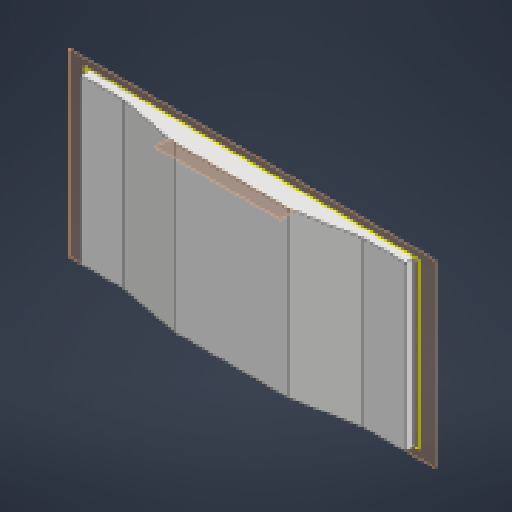
# Autodesk Inventor part: daiza
Saved by Autodesk Inventor 2026.1 (Build 301233020, 233B)
## iProperties
Created: 2026-03-17
Part Number: daiza
Material: 一般
Document SubType Name: Modeling
Designer: kamada
Density: 1 g/cm^3
Appearance: 既定
Author: kamada
Autodesk Inventor part; units mm, degrees
ref_plane "YZ Plane" through (0, 0, 0) normal (1, 0, 0) x (0, 1, 0)
ref_plane "XZ Plane" through (0, 0, 0) normal (0, 1, 0) x (-1, 0, 0)
ref_plane "XY Plane" through (0, 0, 0) normal (0, 0, 1) x (1, 0, 0)
ref_plane "作業平面1" through (0, 0, 0) normal (0, 0, 1) x (1, 0, 0)
ref_plane "作業平面2" through (53.1084, 38.98, 5) normal (0, 1, 0) x (-1, 0, 0)
sketch "スケッチ2" plane through (53.1084, 38.98, 5) normal (0, 1, 0) x (-1, 0, 0)
  line L0 (0, 0) -> (27.0868, 0) projected
  line L1 (27.0868, 0) -> (27.0868, 3) projected
  line L2 (0, 3) -> (27.0868, 3) projected
  line L3 (0, 0) -> (0, 3) projected
  line L4 (53.1084, -5) -> (-26.0192, -5) projected
  line L5 (27.0868, 0) -> (53.1084, -5)
  line L6 (0, 0) -> (-26.0192, -5)
  line L7 (-14.9983, -5) -> (42.0865, -5)
  line L8 (42.0865, -5) -> (42.0865, -2.8822)
  line L9 (42.0865, -2.8822) -> (-14.9983, -2.8822)
  line L10 (-14.9983, -2.8822) -> (-14.9983, -5)
  point P0 (42.0865, -5)
  constraints: 12 end point, 3 point on line, 2 parallel, 1 horizontal, 1 perpendicular
ref_plane "作業平面3" through (-29.3223, 0, -100) normal (0, 1, 0) x (0, 0, 1)
extrude "押し出し1" add sketch "スケッチ2" against normal up to surface (38.98 mm away) contours L0 L5 L9 L6 | L9 L8 L4 L10
sketch "スケッチ3" plane through (68.1068, 38.98, 2.1178) normal (1, 0, 0) x (0, 0, -1)
  line L0 (2.1178, -38.98) -> (0, -38.98) projected
  line L1 (2.1178, 0) -> (2.1178, -38.98) projected
  line L2 (0, 0) -> (2.1178, 0) projected
  line L3 (0, 0) -> (0, -38.98) projected
  point P0 (2.1178, -38.98)
extrude "押し出し2" add sketch "スケッチ3" along normal blind 10
sketch "スケッチ4" plane through (11.0219, 38.98, 0) normal (-1, 0, 0) x (0, 0, 1)
  line L0 (2.1178, -38.98) -> (0, -38.98) projected
  line L1 (2.1178, 0) -> (2.1178, -38.98) projected
  line L2 (0, 0) -> (2.1178, 0) projected
  line L3 (0, 0) -> (0, -38.98) projected
  point P0 (0, -38.98)
extrude "押し出し3" add sketch "スケッチ4" along normal blind 10
sketch "スケッチ5" plane through (78.1068, 0, 0) normal (0, 0, -1) x (-1, 0, 0)
  point P0 (78.1068, 0)
sketch "スケッチ6" plane through (78.1068, 0, 0) normal (0, 0, -1) x (-1, 0, 0)
  line L0 (77.0849, 0) -> (0, 0) projected
  line L1 (44.8216, 0) -> (32.0369, 0)
  line L2 (32.0369, 0) -> (32.0369, 3)
  line L3 (32.0369, 3) -> (44.8216, 3)
  line L4 (44.8216, 3) -> (44.8216, 0)
  point P0 (78.1068, 0)
  dimension "d6" = 3
  constraints: 8 end point, 2 parallel, 1 horizontal, 1 perpendicular, 1 point on line
  measures "d6" distance of L1.end L2.end
extrude "押し出し4" add sketch "スケッチ6" along normal blind 10
sketch "スケッチ7" plane through (26.0216, 0, 5) normal (0, -1, 0) x (1, 0, 0)
  circle A0 centre (13.5428, -12.529) radius 1 projected
  line L0 (-24.9997, -5) -> (7.2636, -5) projected
  line L1 (7.2636, -5) -> (7.2636, -15) projected
  line L2 (20.0483, -15) -> (7.2636, -15) projected
  line L3 (20.0483, -5) -> (20.0483, -15) projected
  line L4 (20.0483, -5) -> (52.0851, -5) projected
  line L5 (52.0851, -2.8822) -> (52.0851, -5) projected
  line L6 (42.0851, -2.8822) -> (52.0851, -2.8822) projected
  line L7 (42.0851, -2.8822) -> (27.0868, 0) projected
  line L8 (27.0868, 0) -> (0, 0) projected
  line L9 (0, 0) -> (-14.9997, -2.8822) projected
  line L10 (-14.9997, -2.8822) -> (-24.9997, -2.8822) projected
  line L11 (-24.9997, -5) -> (-24.9997, -2.8822) projected
  arc A1 (10.5428, -13) -> (7.5428, -10) centre (7.5428, -13) ccw projected
  line L12 (7.5428, -10) -> (-7.2446, -10) projected
  arc A2 (-48.4497, -42.0615) -> (-51.1373, -39.8369) centre (-51.3498, -42.8294) ccw projected
  arc A3 (-51.62, -39.7919) -> (-51.1373, -39.8369) centre (-50.3577, -28.8593) ccw projected
  arc A4 (-51.62, -39.7919) -> (-54.0854, -40.6508) centre (-51.9641, -42.7721) ccw projected
  line L13 (-54.0854, -40.6508) -> (-54.4653, -41.0306) projected
  arc A5 (-54.4653, -41.0306) -> (-55.3439, -43.1519) centre (-52.3439, -43.1519) ccw projected
  line L14 (-55.3439, -43.1519) -> (-55.3439, -50.9664) projected
  arc A6 (-55.3439, -50.9664) -> (-54.4653, -53.0877) centre (-52.3439, -50.9664) ccw projected
  line L15 (-25.2427, -82.3102) -> (-54.4653, -53.0877) projected
  line L16 (-25.2427, -82.3102) -> (-15.2458, -104.9972) projected
  line L17 (-15.2458, -105) -> (-15.2458, -104.9972) projected
  line L18 (42.3302, -105) -> (-15.2458, -105) projected
  line L19 (42.3302, -105) -> (52.3314, -82.3072) projected
  line L20 (81.5522, -53.0864) -> (52.3314, -82.3072) projected
  arc A7 (81.5522, -53.0864) -> (82.4308, -50.9651) centre (79.4308, -50.9651) ccw projected
  line L21 (82.4308, -50.9651) -> (82.4308, -43.1519) projected
  arc A8 (82.4308, -43.1519) -> (81.5522, -41.0306) centre (79.4308, -43.1519) ccw projected
  line L22 (81.5522, -41.0306) -> (81.2592, -40.7377) projected
  arc A9 (81.2592, -40.7377) -> (78.7777, -39.8807) centre (79.1379, -42.859) ccw projected
  arc A10 (78.2031, -39.9351) -> (78.7777, -39.8807) centre (77.4446, -28.8593) ccw projected
  arc A11 (78.2031, -39.9351) -> (75.508, -42.1602) centre (78.408, -42.9281) ccw projected
  line L23 (75.508, -42.1602) -> (74.8779, -44.5397) projected
  arc A12 (74.0992, -45.8932) -> (74.8779, -44.5397) centre (71.9778, -43.7718) ccw projected
  line L24 (74.0992, -45.8932) -> (67.6718, -52.3205) projected
  arc A13 (63.4292, -52.3205) -> (67.6718, -52.3205) centre (65.5505, -50.1992) ccw projected
  line L25 (63.4292, -52.3205) -> (53.9943, -42.8856) projected
  arc A14 (53.9943, -38.643) -> (53.9943, -42.8856) centre (56.1156, -40.7643) ccw projected
  line L26 (53.9943, -38.643) -> (61.0598, -31.5775) projected
  arc A15 (62.5981, -30.756) -> (61.0598, -31.5775) centre (63.1811, -33.6988) ccw projected
  line L27 (62.5981, -30.756) -> (64.1721, -30.4442) projected
  arc A16 (64.1721, -30.4442) -> (66.5799, -27.7364) centre (63.5891, -27.5014) ccw projected
  line L28 (66.7185, -25.9725) -> (66.5799, -27.7364) projected
  line L29 (66.1386, -21.9894) -> (66.7185, -25.9725) projected
  line L30 (66.1386, -21.9894) -> (63.3702, -11.8878) projected
  arc A17 (63.3702, -11.8878) -> (61.2688, -9.7871) centre (60.4769, -12.6807) ccw projected
  ellipse E0 centre (62.8528, -4) end of major axis (56.8528, -4) minor radius 6 (57.9794, -7.5) -> (61.2688, -9.7871) ccw projected
  ellipse E1 centre (53.106, -11) end of major axis (59.106, -11) minor radius 6 (57.9794, -7.5) -> (53.106, -5) ccw projected
  line L31 (-26.0216, -5) -> (53.106, -5) projected
  ellipse E2 centre (-26.0216, -11) end of major axis (-26.0216, -17) minor radius 6 (-26.0216, -5) -> (-30.895, -7.5) ccw projected
  ellipse E3 centre (-35.7684, -4) end of major axis (-35.7684, 2) minor radius 6 (-34.1842, -9.7871) -> (-30.895, -7.5) ccw projected
  arc A18 (-34.1842, -9.7871) -> (-36.2855, -11.8883) centre (-33.392, -12.6806) ccw projected
  line L32 (-36.2855, -11.8883) -> (-39.0518, -21.9905) projected
  line L33 (-39.6698, -26.2352) -> (-39.0518, -21.9905) projected
  ellipse E4 centre (-50.3577, -28.8593) end of major axis (-50.3577, -39.8645) minor radius 11.0053 (-39.4029, -27.806) -> (-39.6698, -26.2352) ccw projected
  arc A19 (-39.4029, -27.806) -> (-36.9997, -30.4616) centre (-36.4167, -27.5188) ccw projected
  line L34 (-36.9997, -30.4616) -> (-35.5138, -30.756) projected
  arc A20 (-33.9754, -31.5775) -> (-35.5138, -30.756) centre (-36.0967, -33.6988) ccw projected
  line L35 (-33.9754, -31.5775) -> (-26.7655, -38.7874) projected
  arc A21 (-26.1405, -42.1163) -> (-26.7655, -38.7874) centre (-28.8868, -40.9087) ccw projected
  line L36 (-26.1405, -42.1163) -> (-26.1393, -42.1175) projected
  line L37 (-26.1393, -42.1175) -> (-37.0994, -53.0777) projected
  line L38 (-37.0994, -53.0777) -> (-37.1007, -53.0764) projected
  arc A22 (-40.4482, -52.4598) -> (-37.1007, -53.0764) centre (-38.3269, -50.3385) ccw projected
  line L39 (-40.4482, -52.4598) -> (-47.0148, -45.8932) projected
  arc A23 (-47.7935, -44.5397) -> (-47.0148, -45.8932) centre (-44.8935, -43.7718) ccw projected
  line L40 (-47.7935, -44.5397) -> (-48.4497, -42.0615) projected
  line L41 (46.4527, -46.6625) -> (59.4096, -59.6194) projected
  arc A24 (59.4096, -63.8621) -> (59.4096, -59.6194) centre (57.2883, -61.7408) ccw projected
  line L42 (59.4096, -63.8621) -> (46.4527, -76.819) projected
  arc A25 (41.3314, -74.6977) -> (46.4527, -76.819) centre (44.3314, -74.6977) ccw projected
  line L43 (41.3314, -74.6977) -> (41.3314, -48.7838) projected
  arc A26 (46.4527, -46.6625) -> (41.3314, -48.7838) centre (44.3314, -48.7838) ccw projected
  line L44 (-19.3659, -77.3873) -> (-32.6069, -64.1463) projected
  arc A27 (-32.6069, -59.9036) -> (-32.6069, -64.1463) centre (-30.4856, -62.025) ccw projected
  line L45 (-32.6069, -59.9036) -> (-19.3659, -46.6626) projected
  arc A28 (-14.2446, -48.7839) -> (-19.3659, -46.6626) centre (-17.2446, -48.7839) ccw projected
  line L46 (-14.2446, -48.7839) -> (-14.2446, -75.266) projected
  arc A29 (-19.3659, -77.3873) -> (-14.2446, -75.266) centre (-17.2446, -75.266) ccw projected
  circle A30 centre (-51.7365, -41.9761) radius 0.75 projected
  circle A31 centre (78.8234, -41.9761) radius 0.75 projected
  line L47 (-7.2446, -100) -> (34.3314, -100) projected
  arc A32 (-10.2446, -97) -> (-7.2446, -100) centre (-7.2446, -97) ccw projected
  line L48 (-10.2446, -13) -> (-10.2446, -97) projected
  arc A33 (-7.2446, -10) -> (-10.2446, -13) centre (-7.2446, -13) ccw projected
  line L49 (7.5428, -10) -> (-7.2446, -10) projected
  arc A34 (10.5428, -13) -> (7.5428, -10) centre (7.5428, -13) ccw projected
  ellipse E5 centre (13.5428, -12.529) end of major axis (13.5428, -15.5657) minor radius 3.0367 (10.5428, -13) -> (11.7776, -15) ccw projected
  line L50 (15.308, -15) -> (11.7776, -15) projected
  ellipse E6 centre (13.5428, -12.529) end of major axis (13.5428, -15.5657) minor radius 3.0367 (15.308, -15) -> (16.5428, -13) ccw projected
  ellipse E7 centre (19.5428, -13) end of major axis (16.5428, -13) minor radius 3 (19.5428, -10) -> (16.5428, -13) ccw projected
  line L51 (34.3314, -10) -> (19.5428, -10) projected
  arc A35 (37.3314, -13) -> (34.3314, -10) centre (34.3314, -13) ccw projected
  line L52 (37.3314, -97) -> (37.3314, -13) projected
  arc A36 (34.3314, -100) -> (37.3314, -97) centre (34.3314, -97) ccw projected
  circle A37 centre (49.6906, -42.1175) radius 1.05 projected
  circle A38 centre (64.1863, -56.6132) radius 1.05 projected
  circle A39 centre (64.3278, -27.4804) radius 1.05 projected
  circle A40 centre (13.5428, -12.529) radius 1 projected
  circle A41 centre (49.6905, -10.0007) radius 1.05 projected
  circle A42 centre (-37.2408, -27.4804) radius 1.05 projected
  circle A43 centre (-22.6037, -42.1175) radius 1.05 projected
  circle A44 centre (-37.0994, -56.6132) radius 1.05 projected
  circle A45 centre (-22.6052, -10.0012) radius 1.05 projected
  line L53 (-15.2446, -20.5845) -> (-15.2446, -31.5342) projected
  arc A46 (-15.8673, -33.3641) -> (-15.2446, -31.5342) centre (-18.2446, -31.5342) ccw projected
  line L54 (-15.8673, -33.3641) -> (-16.1001, -33.6665) projected
  arc A47 (-18.4774, -34.8367) -> (-16.1001, -33.6665) centre (-18.4774, -31.8367) ccw projected
  line L55 (-18.4774, -34.8367) -> (-19.7435, -34.8367) projected
  arc A48 (-21.882, -33.9406) -> (-19.7435, -34.8367) centre (-19.7435, -31.8367) ccw projected
  line L56 (-21.882, -33.9406) -> (-31.4665, -24.1986) projected
  arc A49 (-32.3279, -22.0947) -> (-31.4665, -24.1986) centre (-29.3279, -22.0947) ccw projected
  line L57 (-32.3279, -22.0947) -> (-32.3279, -18.6116) projected
  arc A50 (-31.7009, -16.776) -> (-32.3279, -18.6116) centre (-29.3279, -18.6116) ccw projected
  line L58 (-31.7009, -16.776) -> (-31.2287, -16.1656) projected
  arc A51 (-28.8558, -15.0012) -> (-31.2287, -16.1656) centre (-28.8558, -18.0012) ccw projected
  line L59 (-28.8558, -15.0012) -> (-20.2331, -15.0012) projected
  arc A52 (-17.8558, -16.1713) -> (-20.2331, -15.0012) centre (-20.2331, -18.0012) ccw projected
  line L60 (-17.8558, -16.1713) -> (-15.8673, -18.7546) projected
  arc A53 (-15.2446, -20.5845) -> (-15.8673, -18.7546) centre (-18.2446, -20.5845) ccw projected
  line L61 (42.3314, -31.535) -> (42.3314, -20.5837) projected
  arc A54 (42.954, -18.754) -> (42.3314, -20.5837) centre (45.3314, -20.5837) ccw projected
  line L62 (42.954, -18.754) -> (44.9417, -16.1714) projected
  arc A55 (47.3191, -15.0012) -> (44.9417, -16.1714) centre (47.3191, -18.0012) ccw projected
  line L63 (47.3191, -15.0012) -> (55.8745, -15.0012) projected
  arc A56 (58.2474, -16.1656) -> (55.8745, -15.0012) centre (55.8745, -18.0012) ccw projected
  line L64 (58.2474, -16.1656) -> (58.7196, -16.776) projected
  arc A57 (59.3466, -18.6116) -> (58.7196, -16.776) centre (56.3466, -18.6116) ccw projected
  line L65 (59.3466, -18.6116) -> (59.3466, -22.099) projected
  arc A58 (58.4904, -24.1977) -> (59.3466, -22.099) centre (56.3466, -22.099) ccw projected
  line L66 (58.4904, -24.1977) -> (48.9577, -33.9353) projected
  arc A59 (46.8139, -34.8367) -> (48.9577, -33.9353) centre (46.8139, -31.8367) ccw projected
  line L67 (46.8139, -34.8367) -> (45.5636, -34.8367) projected
  arc A60 (43.1862, -33.6664) -> (45.5636, -34.8367) centre (45.5636, -31.8367) ccw projected
  line L68 (43.1862, -33.6664) -> (42.954, -33.3647) projected
  arc A61 (42.3314, -31.535) -> (42.954, -33.3647) centre (45.3314, -31.535) ccw projected
  circle A62 centre (-17.6082, -89.4172) radius 1 projected
  circle A63 centre (40.0144, -102.2006) radius 1 projected
  circle A64 centre (-12.93, -102.2006) radius 1 projected
  circle A65 centre (44.6926, -89.4172) radius 1 projected
  point P0 (-26.0216, -5)
  point P1 (7.2636, -10)
  point P2 (20.0483, -10)
  constraints: 8 other
extrude "押し出し5" cut sketch "スケッチ7" against normal blind 10 contours L12 A1 E5 L2 L1 | L3 L2 E6 E7 L51
fillet "フィレット1" radius 2 3 edges at (46.0699, 1.5, 0) (33.2852, 1.5, 0) (39.6775, 3, 0)
sketch "スケッチ8" plane through (1.0219, 38.98, 2.1178) normal (0, 0, 1) x (1, 0, 0)
  line L0 (4, -5) -> (73.0849, -5)
  line L1 (73.0849, -5) -> (73.0849, -33.98)
  line L2 (73.0849, -33.98) -> (4, -33.98)
  line L3 (4, -33.98) -> (4, -5)
  line L4 (0, -38.98) -> (0, 0) projected
  line L5 (77.0849, 0) -> (77.0849, -38.98) projected
  line L6 (10, -38.98) -> (0, -38.98) projected
  line L7 (10, 0) -> (0, 0) projected
  circle A0 centre (73.0849, -5) radius 1
  circle A1 centre (73.0849, -33.98) radius 1
  circle A2 centre (4, -33.98) radius 1
  circle A3 centre (4, -5) radius 1
  point P0 (-1.0219, -38.98)
  point P1 (4, -19.49)
  point P2 (0, -19.49)
  point P3 (77.0849, -19.49)
  dimension "d12" = 4
  dimension "d13" = 4
  dimension "d14" = 5
  dimension "d15" = 5
  dimension "d16" = 2
  dimension "d17" = 2
  dimension "d18" = 2
  dimension "d19" = 2
  constraints: 8 end point, 4 centre point, 4 coincident, 3 midpoint, 2 parallel, 1 horizontal, 1 perpendicular
  measures "d12" distance of point (4, -19.49) point (0, -19.49)
  measures "d13" distance from line of point (77.085, -19.49) L1
  measures "d14" distance between parallel lines of L6 L2
  measures "d15" distance between parallel lines of L7 L0
  measures "d16" diameter of A0
  measures "d17" diameter of A1
  measures "d18" diameter of A2
  measures "d19" diameter of A3
extrude "押し出し6" cut sketch "スケッチ8" against normal blind 10 contours L3 A3 L0 | L0 A3 L3 | A0 L1 L0 | L0 L1 A0 | A2 L2 L3 | L3 L2 A2 | A1 L2 L1 | L1 L2 A1
ref_plane "作業平面4" through (0, 0, 0) normal (0, 0, 1) x (1, 0, 0)
sketch "スケッチ9" plane through (0, 0, 0) normal (0, 0, 1) x (1, 0, 0)
  circle A0 centre (5.0219, 5) radius 1 projected
  circle A1 centre (5.0219, 33.98) radius 1 projected
  circle A2 centre (74.1068, 33.98) radius 1 projected
  circle A3 centre (74.1068, 5) radius 1 projected
  point P0 (0, 0)
sketch "スケッチ10" plane through (26.0216, 38.98, 5) normal (0, 0, 1) x (1, 0, 0)
  circle A0 centre (3.5807, -27.6915) radius 1 projected
  circle A1 centre (23.5061, -27.6915) radius 1 projected
  circle A2 centre (23.5061, -4.9192) radius 1 projected
  circle A3 centre (3.5807, -4.9192) radius 1 projected
  arc A4 (18.5347, -17) -> (13.5434, -11.7052) centre (13.5434, -16.7052) ccw projected
  circle A5 centre (13.5434, -16.7052) radius 5
  point P0 (-26.0216, -38.98)
  point P1 (18.5347, -17)
  constraints: 1 centre point, 1 coincident, 1 concentric
extrude "押し出し7" cut sketch "スケッチ10" against normal blind 10
sketch "スケッチ11" plane through (26.0216, 0, 5) normal (0, -1, 0) x (1, 0, 0)
  circle A0 centre (13.5428, -12.529) radius 1 projected
  point P0 (-26.0216, -5)
extrude "押し出し8" cut sketch "スケッチ11" against normal blind 10
sketch "スケッチ12" plane through (37.7992, 3, -10) normal (0, 1, 0) x (1, 0, 0)
  circle A0 centre (1.7652, -2.471) radius 1 projected
  line L0 (2.9776, -0.371) -> (4.1901, -2.471)
  line L1 (4.1901, -2.471) -> (2.9776, -4.571)
  line L2 (2.9776, -4.571) -> (0.5528, -4.571)
  line L3 (0.5528, -4.571) -> (-0.6597, -2.471)
  line L4 (-0.6597, -2.471) -> (0.5528, -0.371)
  line L5 (0.5528, -0.371) -> (2.9776, -0.371)
  point P0 (-37.7992, -10)
  dimension "d26" = 4.2
  constraints: 12 end point, 1 coincident, 13 other
  measures "d26" distance between parallel lines of L5 L2
extrude "押し出し9" cut sketch "スケッチ12" against normal blind 2 contours A0 | L0 L1 L2 L3 L4 L5
fillet "フィレット2" radius 2 2 edges at (33.2852, 1.5, -5) (46.0699, 1.5, -5)
sketch "スケッチ13" plane through (78.1068, 0, 0) normal (0, 0, -1) x (-1, 0, 0)
  circle A0 centre (48.5045, 11.2885) radius 1 projected
  circle A1 centre (48.5045, 34.0608) radius 1 projected
  circle A2 centre (28.579, 11.2885) radius 1 projected
  circle A3 centre (28.579, 34.0608) radius 1 projected
  circle A4 centre (38.5417, 22.2748) radius 5 projected
  circle A5 centre (4, 5) radius 1 projected
  circle A6 centre (73.0849, 5) radius 1 projected
  circle A7 centre (4, 33.98) radius 1 projected
  circle A8 centre (73.0849, 33.98) radius 1 projected
  line L0 (30.0369, 5) -> (30.0369, 0) projected
  line L1 (46.8216, 5) -> (30.0369, 5) projected
  line L2 (46.8216, 0) -> (46.8216, 5) projected
  line L3 (77.0849, 0) -> (46.8216, 0) projected
  line L4 (77.0849, 38.98) -> (77.0849, 0) projected
  line L5 (0, 38.98) -> (77.0849, 38.98) projected
  line L6 (0, 0) -> (0, 38.98) projected
  line L7 (30.0369, 0) -> (0, 0) projected
  line L8 (29.7914, 36.1608) -> (31.0039, 34.0608)
  line L9 (31.0039, 34.0608) -> (29.7914, 31.9608)
  line L10 (29.7914, 31.9608) -> (27.3666, 31.9608)
  line L11 (27.3666, 31.9608) -> (26.1541, 34.0608)
  line L12 (26.1541, 34.0608) -> (27.3666, 36.1608)
  line L13 (27.3666, 36.1608) -> (29.7914, 36.1608)
  line L14 (49.7169, 36.1608) -> (50.9293, 34.0608)
  line L15 (50.9293, 34.0608) -> (49.7169, 31.9608)
  line L16 (49.7169, 31.9608) -> (47.292, 31.9608)
  line L17 (47.292, 31.9608) -> (46.0796, 34.0608)
  line L18 (46.0796, 34.0608) -> (47.292, 36.1608)
  line L19 (47.292, 36.1608) -> (49.7169, 36.1608)
  line L20 (49.7169, 13.3885) -> (50.9293, 11.2885)
  line L21 (50.9293, 11.2885) -> (49.7169, 9.1885)
  line L22 (49.7169, 9.1885) -> (47.292, 9.1885)
  line L23 (47.292, 9.1885) -> (46.0796, 11.2885)
  line L24 (46.0796, 11.2885) -> (47.292, 13.3885)
  line L25 (47.292, 13.3885) -> (49.7169, 13.3885)
  line L26 (29.7914, 13.3885) -> (31.0039, 11.2885)
  line L27 (31.0039, 11.2885) -> (29.7914, 9.1885)
  line L28 (29.7914, 9.1885) -> (27.3666, 9.1885)
  line L29 (27.3666, 9.1885) -> (26.1541, 11.2885)
  line L30 (26.1541, 11.2885) -> (27.3666, 13.3885)
  line L31 (27.3666, 13.3885) -> (29.7914, 13.3885)
  point P0 (78.1068, 0)
  point P1 (48.5045, 36.1608)
  point P2 (28.579, 31.9608)
  point P3 (48.5045, 31.9608)
  point P4 (28.579, 9.1885)
  point P5 (28.579, 13.3885)
  dimension "d30" = 4.2
  dimension "d31" = 4.2
  dimension "d32" = 4.2
  dimension "d33" = 4.2
  constraints: 48 end point, 5 midpoint, 4 coincident, 3 equal length, 1 point on line, 52 other
  measures "d30" distance from line of point (28.579, 31.961) L13
  measures "d31" distance from line of point (48.504, 31.961) L19
  measures "d32" distance between parallel lines of L22 L25
  measures "d33" distance of point (28.579, 9.188) point (28.579, 13.388)
extrude "押し出し10" cut sketch "スケッチ13" against normal blind 2.2 contours A0 | A1 | A2 | A3 | L8 L9 L10 L11 L12 L13 | L14 L15 L16 L17 L18 L19 | L20 L21 L22 L23 L24 L25 | L26 L27 L28 L29 L30 L31
fillet "フィレット3" radius 0.2 24 edges at (51.3464, 33.0108, 0) (51.3464, 35.1108, 0) (49.5278, 36.1608, 0) (47.7091, 35.1108, 0) (47.7091, 33.0108, 0) (49.5278, 31.9608, 0) (29.6023, 31.9608, 0) (27.7837, 33.0108, 0) (27.7837, 35.1108, 0) (29.6023, 36.1608, 0) (31.421, 35.1108, 0) (31.421, 33.0108, 0) (31.421, 12.3385, 0) (29.6023, 13.3885, 0) (27.7837, 12.3385, 0) (27.7837, 10.2385, 0) (29.6023, 9.1885, 0) (31.421, 10.2385, 0) (51.3464, 12.3385, 0) (49.5278, 13.3885, 0) (47.7091, 12.3385, 0) (47.7091, 10.2385, 0) (49.5278, 9.1885, 0) (51.3464, 10.2385, 0)
fillet "フィレット4" radius 1 1 edges at (34.5737, 22.5695, 0)
equation "\"d12\" = d13"
equation "\"d15\" = d14"
equation "\"d31\" = d30"
equation "\"d32\" = d31"
equation "\"d33\" = d32"
